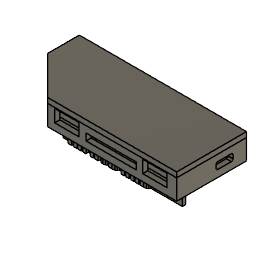
USB HUB assembly (Autodesk Fusion 360 design; units mm, degrees)
part number: 2026-07-31-23-58-47-749
Autodesk Fusion 360 part; units mm, degrees
note: some values were not read from the file. Set by a fixed rule: which sketch regions a step uses.
sketch "Sketch1" plane through (0, 0, 0) normal (0, 0, 1) x (1, 0, 0)
  line L0 (-50, 50) -> (40, 50)
  line L1 (40, 50) -> (40, 17)
  line L2 (40, 17) -> (-30, 17)
  line L3 (-50, 37) -> (-50, 50)
  line L4 (40, 17) -> (-30, 17)
  line L5 (-50, 50) -> (-50, 37)
  line L6 (-50, 37) -> (-30, 17)
  line L7 (-51, 36.5858) -> (-30.4142, 16)
  line L8 (41, 16) -> (-30.4142, 16)
  line L9 (41, 51) -> (41, 16)
  line L10 (-51, 51) -> (41, 51)
  line L11 (-51, 51) -> (-51, 36.5858)
  line L12 (44, 13) -> (-31.6569, 13)
  line L13 (-54, 35.3431) -> (-31.6569, 13)
  line L14 (-54, 54) -> (-54, 35.3431)
  line L15 (-54, 54) -> (44, 54)
  line L16 (44, 54) -> (44, 13)
  dimension "d2" = 90
  dimension "d3" = 70
  dimension "d4" = 13
  dimension "d5" = -1
  dimension "d6" = -3
  constraint horizontal L0
  constraint vertical L1
  constraint horizontal L2
  constraint vertical L3
  measures "d2" distance of L0.start L0.end
  measures "d3" distance of L1.end L2.end
  measures "d4" distance of L0.start L3.start
extrude "Extrude1" add sketch "Sketch1" along normal blind 10.9 contours L12 L13 L14 L15 L16 makes body 1
extrude "Extrude2" add 1 faces at (-20.3333, 53, 10.9) along direction (0, 0, 1) blind 1 on bodies 1 bodies 1
extrude "Extrude3" add sketch "Sketch1" along normal blind 3 contours L0 L1 L2 L3 L4 L5 L6 | L7 L8 L9 L10 L11 bodies 1
sketch "Sketch2" plane through (0, 17, 0) normal (0, -1, 0) x (1, 0, 0)
  line L0 (-30, 3) -> (40, 3)
  line L1 (40, 3) -> (40, 10.9)
  line L2 (40, 10.9) -> (-30, 10.9)
  line L3 (-30, 10.9) -> (-30, 3)
  line L4 (-30, 3) -> (-26.95, 3)
  line L5 (-26.95, 3) -> (-26.95, 4.6)
  line L6 (-26.95, 4.6) -> (-13.75, 4.6)
  line L7 (-13.75, 4.6) -> (-13.75, 10.9)
  line L8 (-13.75, 10.9) -> (-26.95, 10.9)
  line L9 (-26.95, 10.9) -> (-26.95, 4.6)
  line L10 (-30, 3) -> (24.6, 3)
  line L11 (24.6, 3) -> (24.6, 4.6)
  line L12 (24.6, 4.6) -> (37.8, 4.6)
  line L13 (37.8, 4.6) -> (37.8, 10.9)
  line L14 (37.8, 10.9) -> (24.6, 10.9)
  line L15 (24.6, 10.9) -> (24.6, 4.6)
  line L16 (-30, 3) -> (-8.6, 3)
  line L17 (-8.6, 3) -> (-8.6, 4.6)
  line L18 (-8.6, 4.6) -> (19.9, 4.6)
  line L19 (19.9, 4.6) -> (19.9, 7.6)
  line L20 (19.9, 7.6) -> (-8.6, 7.6)
  line L21 (-8.6, 7.6) -> (-8.6, 4.6)
  line L22 (-27.45, 4.1) -> (-13.25, 4.1)
  line L23 (-13.25, 4.1) -> (-13.25, 11.4)
  line L24 (-13.25, 11.4) -> (-27.45, 11.4)
  line L25 (-27.45, 11.4) -> (-27.45, 4.1)
  line L26 (-9.1, 4.1) -> (20.4, 4.1)
  line L27 (20.4, 4.1) -> (20.4, 8.1)
  line L28 (20.4, 8.1) -> (-9.1, 8.1)
  line L29 (-9.1, 8.1) -> (-9.1, 4.1)
  line L30 (38.3, 4.1) -> (38.3, 11.4)
  line L31 (38.3, 11.4) -> (24.1, 11.4)
  line L32 (24.1, 11.4) -> (24.1, 4.1)
  line L33 (24.1, 4.1) -> (38.3, 4.1)
  dimension "d15" = 3.05
  dimension "d16" = 1.6
  dimension "d17" = 6.3
  dimension "d18" = 13.2
  dimension "d19" = 54.6
  dimension "d20" = 1.6
  dimension "d21" = 6.3
  dimension "d22" = 13.2
  dimension "d23" = 21.4
  dimension "d24" = 1.6
  dimension "d25" = 3
  dimension "d26" = 28.5
  dimension "d27" = 0.5
  dimension "d28" = 0.5
  dimension "d29" = 0.5
  constraint coincident L0.start L3.end
  constraint perpendicular L3 L4
  constraint perpendicular L4 L5
  constraint horizontal L6
  constraint vertical L7
  constraint horizontal L8
  constraint vertical L9
  constraint perpendicular L3 L10
  constraint perpendicular L10 L11
  constraint horizontal L12
  constraint vertical L13
  constraint horizontal L14
  constraint vertical L15
  constraint coincident L2 L13.end
  constraint parallel L10 L16
  constraint perpendicular L0 L17
  constraint horizontal L18
  constraint vertical L19
  constraint horizontal L20
  constraint vertical L21
  measures "d15" distance of L0.start L4.end
  measures "d16" distance of L4.end L5.end
  measures "d17" distance of L5.end L8.end
  measures "d18" distance of L5.end L6.end
  measures "d19" distance of L0.start L10.end
  measures "d20" distance of L10.end L11.end
  measures "d21" distance of L11.end L14.end
  measures "d22" distance of L11.end L12.end
  measures "d23" distance of L0.start L16.end
  measures "d24" distance of L16.end L17.end
  measures "d25" distance of L17.end L20.end
  measures "d26" distance of L17.end L18.end
extrude "Extrude5" cut sketch "Sketch2" along normal blind 13 contours L2 L5 L9 L22 L25 | L2 L5 L6 L7 L22 L23 | L2 L8 L23 L24 L25 | L2 L6 L7 L8 L9 | L2 L11 L15 L32 L33 | L2 L11 L12 L13 L30 L33 | L2 L12 L13 L14 L15 | L2 L14 L30 L31 L32 | L18 L19 L20 L21 | L26 L27 L28 L29 bodies 1
sketch "Sketch3" plane through (40, 0, 0) normal (1, 0, 0) x (0, 1, 0)
  line L0 (17, 3) -> (50, 3)
  line L1 (50, 3) -> (50, 10.9)
  line L2 (50, 10.9) -> (17, 10.9)
  line L3 (17, 10.9) -> (17, 3)
  line L4 (17, 3) -> (17, 4.6)
  line L5 (17, 4.6) -> (45.1, 4.6)
  line L6 (50, 4.6) -> (50, 3)
  line L7 (36.6, 5.1) -> (36.6, 7.1)
  line L8 (37.1, 7.6) -> (45.1, 7.6)
  line L9 (45.6, 7.1) -> (45.6, 5.1)
  arc A0 (37.1, 7.6) -> (36.6, 7.1) centre (37.1, 7.1) ccw
  arc A1 (45.6, 7.1) -> (45.1, 7.6) centre (45.1, 7.1) ccw
  arc A2 (36.6, 5.1) -> (37.1, 4.6) centre (37.1, 5.1) ccw
  arc A3 (45.1, 4.6) -> (45.6, 5.1) centre (45.1, 5.1) ccw
  line L10 (17.5, 3) -> (17.5, 4.1)
  line L11 (17.5, 4.1) -> (37.1, 4.1)
  line L12 (37.1, 4.1) -> (45.1, 4.1)
  arc A4 (45.1, 4.1) -> (46.1, 5.1) centre (45.1, 5.1) ccw
  line L13 (46.1, 7.1) -> (46.1, 5.1)
  arc A5 (46.1, 7.1) -> (45.1, 8.1) centre (45.1, 7.1) ccw
  line L14 (37.1, 8.1) -> (45.1, 8.1)
  arc A6 (37.1, 8.1) -> (36.1, 7.1) centre (37.1, 7.1) ccw
  line L15 (36.1, 5.1) -> (36.1, 7.1)
  arc A7 (36.1, 5.1) -> (37.1, 4.1) centre (37.1, 5.1) ccw
  point P0 (45.6, 7.6)
  dimension "d32" = 1.6
  dimension "d36" = 0.5
  dimension "d37" = -0.5
  constraint coincident L0.start L3.end
  constraint perpendicular L0 L4
  constraint coincident L1 L6.start
  constraint perpendicular L1 L5
  constraint coincident L0.end L1.start
  constraint vertical L7
  constraint horizontal L8
  constraint vertical L9
  constraint tangent L7 A0
  constraint tangent L8 A0
  constraint coincident P0 L8
  constraint coincident P0 L9
  constraint tangent L8 A1
  constraint tangent L9 A1
  constraint equal A0 A1
  constraint tangent L7 A2
  constraint equal A0 A2
  constraint coincident L6.start L5
  constraint tangent L9 A3
  constraint tangent L5 A3
  constraint equal A0 A3
  measures "d32" distance of L0.start L4.end
  measures "d36" radius of A0
extrude "Extrude6" cut sketch "Sketch3" along normal blind 7 contours L12 A4 L13 A5 L14 A6 L15 A7 | L5 L7 L8 L9 A0 A1 A2 A3 bodies 1
sketch "Sketch4" plane through (-50, 0, 0) normal (-1, 0, 0) x (0, -1, 0)
  line L0 (-50, 3) -> (-37, 3)
  line L1 (-37, 3) -> (-37, 10.9)
  line L2 (-37, 10.9) -> (-50, 10.9)
  line L3 (-50, 10.9) -> (-50, 3)
  line L4 (-50, 3) -> (-50, 4.6)
  line L5 (-50, 3) -> (-48.08, 3)
  line L6 (-50, 4.6) -> (-37, 4.6)
  line L7 (-48.08, 3) -> (-48.08, 4.6)
  line L8 (-47.58, 4.6) -> (-39.58, 4.6)
  line L9 (-39.08, 5.1) -> (-39.08, 7.1)
  line L10 (-39.58, 7.6) -> (-47.58, 7.6)
  line L11 (-48.08, 7.1) -> (-48.08, 5.1)
  arc A0 (-47.58, 7.6) -> (-48.08, 7.1) centre (-47.58, 7.1) ccw
  arc A1 (-39.08, 7.1) -> (-39.58, 7.6) centre (-39.58, 7.1) ccw
  arc A2 (-39.58, 4.6) -> (-39.08, 5.1) centre (-39.58, 5.1) ccw
  arc A3 (-48.08, 5.1) -> (-47.58, 4.6) centre (-47.58, 5.1) ccw
  line L12 (-48.58, 7.1) -> (-48.58, 5.1)
  arc A4 (-48.58, 5.1) -> (-47.58, 4.1) centre (-47.58, 5.1) ccw
  line L13 (-47.58, 4.1) -> (-39.58, 4.1)
  arc A5 (-39.58, 4.1) -> (-38.58, 5.1) centre (-39.58, 5.1) ccw
  line L14 (-38.58, 5.1) -> (-38.58, 7.1)
  arc A6 (-38.58, 7.1) -> (-39.58, 8.1) centre (-39.58, 7.1) ccw
  line L15 (-39.58, 8.1) -> (-47.58, 8.1)
  arc A7 (-47.58, 8.1) -> (-48.58, 7.1) centre (-47.58, 7.1) ccw
  point P0 (-39.08, 7.6)
  point P1 (-48.08, 7.6)
  dimension "d40" = 1.6
  dimension "d41" = 1.92
  dimension "d42" = 3
  dimension "d43" = 9
  dimension "d44" = 0.5
  dimension "d45" = 0.5
  constraint coincident L0.start L3.end
  constraint perpendicular L0 L4
  constraint perpendicular L4 L5
  constraint perpendicular L4 L6
  constraint coincident L6 L7.end
  constraint perpendicular L6 L7
  constraint horizontal L8
  constraint vertical L9
  constraint horizontal L10
  constraint vertical L11
  constraint coincident P1 L10
  constraint coincident P1 L11
  constraint tangent L10 A0
  constraint tangent L11 A0
  constraint coincident P0 L9
  constraint coincident P0 L10
  constraint tangent L9 A1
  constraint tangent L10 A1
  constraint equal A0 A1
  constraint tangent L8 A2
  constraint tangent L9 A2
  constraint equal A0 A2
  constraint coincident L7.end L8
  constraint coincident L7.end L11
  constraint tangent L8 A3
  constraint tangent L11 A3
  constraint equal A0 A3
  measures "d40" distance of L0.start L4.end
  measures "d41" distance of L0.start L5.end
  measures "d42" distance of L7.end P1
  measures "d43" distance of P0 P1
  measures "d44" radius of A0
extrude "Extrude7" cut sketch "Sketch4" along normal blind 5 contours L6 L7 A4 | L6 L7 L8 A4 L13 A5 | L6 L9 L10 L11 A0 A1 A2 A3 L12 A4 A5 L14 A6 L15 A7 | L6 L8 L9 L10 L11 A0 A1 A2 A3 bodies 1
extrude "Extrude8" add sketch "Sketch1" along normal blind 3 from surface at 11.9 separate body contours L0 L1 L2 L3 L4 L5 L6 | L7 L8 L9 L10 L11 | L12 L13 L14 L15 L16 makes body 2
sketch "Sketch5" plane through (0, 0, 0) normal (0, 0, -1) x (1, 0, 0)
  line L0 (-54, -35.3431) -> (-54, -54)
  line L1 (-54, -54) -> (44, -54)
  line L2 (44, -54) -> (44, -13)
  line L3 (44, -13) -> (-31.6569, -13)
  line L4 (-31.6569, -13) -> (-54, -35.3431)
  line L5 (44, -13) -> (44, -54)
  line L6 (44, -13) -> (44, -24)
  line L7 (44, -24) -> (-31, -24)
  line L8 (-31.6569, -13) -> (44, -13)
  line L9 (-31.6569, -13) -> (-31.6569, -24)
  line L10 (-31.6569, -24) -> (-31, -24)
  line L11 (-31.6569, -24) -> (38.3431, -24)
  line L12 (38.3431, -24) -> (38.3431, -22)
  line L13 (38.3431, -22) -> (-31.6569, -22)
  line L14 (-31.6569, -22) -> (-31.6569, -24)
  dimension "d51" = 2
  dimension "d52" = 70
  constraint coincident L2.end L3.start
  constraint coincident L1.end L2.start
  constraint coincident L2 L6.end
  constraint perpendicular L5 L7
  constraint coincident L3.end L4.start
  constraint perpendicular L8 L9
  constraint horizontal L11
  constraint vertical L12
  constraint horizontal L13
  constraint vertical L14
  measures "d51" distance of L9.end L13.end
  measures "d52" distance of L12.end L13.end
extrude "Extrude9" add sketch "Sketch5" along normal blind 10 contours L7 L9 L10 L11 L12 L13 L14 bodies 1
sketch "Sketch6" plane through (0, 0, 0) normal (0, 0, -1) x (1, 0, 0)
  line L0 (-31.6569, -22) -> (38.3431, -22)
  line L1 (38.3431, -22) -> (38.3431, -24)
  line L2 (38.3431, -24) -> (-31.6569, -24)
  line L3 (-31.6569, -24) -> (-31.6569, -22)
  line L4 (-54, -35.3431) -> (-54, -54)
  line L5 (-54, -54) -> (44, -54)
  line L6 (44, -54) -> (44, -13)
  line L7 (44, -13) -> (-31.6569, -13)
  line L8 (-31.6569, -13) -> (-54, -35.3431)
  line L9 (-31.6569, -22) -> (38.3409, -22) construction
  line L10 (38.3409, -22) -> (38.3409, -13) construction
  line L11 (38.3409, -13) -> (-31.6569, -13) construction
  line L12 (-31.6569, -13) -> (-31.6569, -22) construction
  dimension "d55" = 8
  text T0 "VK USB HUB" font "Impact" height 8 align centre middle in box 69.9977 x 9 at (-31.6569, -22) x (1, 0) y (0, 1) spacing 1
  constraint coincident L7
  constraint coincident L0.start
extrude "Extrude10" add sketch "Sketch6" along normal blind 3 text T0 bodies 1
extrude "Extrude11" add sketch "Sketch1" along normal blind 1.6 from surface at 3 separate body contours L0 L1 L2 L3 L4 L5 L6 makes body 3
equation "d56 = 'VK USB HUB'"
named bodies: "Case", "Cover", "PCB"
